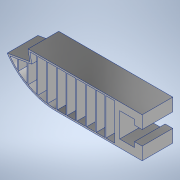
# Autodesk Inventor part: Finray_9_Kerbe_10deg
Saved by Autodesk Inventor 2022 (Build 260153000, 153)
## iProperties
Created: 2022-02-28
Part Number: Finray_9_Kerbe_10deg
Material: Generic
Document SubType Name: Modeling
Designer: richa
Density: 1 g/cm^3
Appearance: Aluminum - Flat
Author: richa
Autodesk Inventor part; units mm, degrees
ref_plane "YZ Plane" through (0, 0, 0) normal (1, 0, 0) x (0, 1, 0)
ref_plane "XZ Plane" through (0, 0, 0) normal (0, 1, 0) x (-1, 0, 0)
ref_plane "XY Plane" through (0, 0, 0) normal (0, 0, 1) x (1, 0, 0)
sketch "Sketch5" plane through (0, 0, 0) normal (0, 0, 1) x (1, 0, 0)
  line L0 (52.8, -15.6) -> (52.8, -10.6)
  line L1 (52.8, -10.6) -> (49.8, -10.6)
  line L2 (49.8, -10.6) -> (49.8, -12.6)
  line L3 (44, -12.6) -> (44, -3)
  line L4 (49.8, -3) -> (49.8, -5)
  line L5 (49.8, -5) -> (52.8, -5)
  line L6 (52.8, -5) -> (52.8, 0)
  line L7 (52.8, 0) -> (7.8, 0)
  line L8 (44, -3) -> (49.8, -3)
  line L9 (44, -12.6) -> (49.8, -12.6)
  line L10 (52.8, -15.6) -> (7.8, -15.6)
  line L11 (7.8, -15.6) -> (0, -15.6)
  line L12 (0, -15.6) -> (0, 0)
  line L13 (0, 0) -> (7.8, 0)
  point P0 (7.8, 0)
  dimension "d41" = 5.8
  dimension "d48" = 44
  dimension "d50" = 3
  dimension "d63" = 45
  dimension "d71" = 0
  dimension "d87" = 5.6
  dimension "d88" = 9.6
  dimension "d97" = 15.6
  constraints: 28 end point, 8 perpendicular, 4 collinear, 3 parallel, 2 horizontal, 1 vertical
  measures "d41" distance between parallel lines of L2 L3
  measures "d48" distance from line of L3 L12.end
  measures "d50" distance of L4.end L5.end
  measures "d63" distance of L0.start L10.end
  measures "d71" distance from line of L12.end L7
  measures "d87" distance from line of L0.end L5
  measures "d88" distance of L3.start L3.end
  measures "d97" distance of L11.end L12.end
extrude "Extrusion2" add sketch "Sketch5" along normal blind 12
sketch "Sketch8" plane through (0, 0, 0) normal (0, 0, -1) x (-1, 0, 0)
  line L0 (-8.1687, 0) -> (-8.8633, -3.9392)
  line L1 (-7.8, 0) -> (-1.143, 0) construction
  line L2 (0, -5.5021) -> (-8.8633, -3.9392)
  line L3 (-7.8, 0) -> (-8.1687, 0)
  line L4 (0, 0) -> (0, -15.6) projected
  line L5 (-52.8, 0) -> (0, 0) projected
  line L6 (-7.8, 0) -> (0, 0)
  line L7 (0, 0) -> (0, -5.5021)
  dimension "d80" = 100
  dimension "d95" = 4
  dimension "d96" = 9
  constraints: 12 end point, 2 collinear, 2 perpendicular, 1 horizontal, 1 point on line
  measures "d80" angle of L0 L1
  measures "d95" distance of L0.start L0.end
  measures "d96" distance of L2.start L0.end
extrude "Extrusion5" cut sketch "Sketch8" against normal through all
fillet "Fillet2" radius 23 1 edges at (0, -15.6, 6)
shell "Shell1" thickness 0.62 removed faces 1 at (23.9679, -7.5131, 12)
sketch "Sketch13" plane through (0, 0, 12) normal (0, 0, 1) x (1, 0, 0)
  line L0 (19.0404, -15.6) -> (52.8, -15.6) projected
  line L1 (42.0526, -15.6) -> (42.0526, 0)
  line L2 (52.8, 0) -> (8.1687, 0) projected
  line L3 (52.8, 0) -> (8.1687, 0) projected
  line L4 (52.8, -5) -> (52.8, 0) projected
  line L5 (49.8, -5) -> (52.8, -5) projected
  line L6 (49.8, -3) -> (49.8, -5) projected
  line L7 (44, -3) -> (49.8, -3) projected
  line L8 (44, -12.6) -> (44, -3) projected
  line L9 (49.8, -12.6) -> (44, -12.6) projected
  line L10 (49.8, -10.6) -> (49.8, -12.6) projected
  line L11 (52.8, -10.6) -> (49.8, -10.6) projected
  line L12 (52.8, -15.6) -> (52.8, -10.6) projected
  line L13 (42.0526, 0) -> (52.8, 0)
  line L14 (52.8, -5) -> (52.8, 0) projected
  line L15 (52.8, -5) -> (52.8, 0)
  line L16 (52.8, 0) -> (52.8, -5)
  line L17 (44, -12.6) -> (44, -3) projected
  line L18 (44, -3) -> (44, -12.6)
  line L19 (49.8, -12.6) -> (44, -12.6) projected
  line L20 (44, -12.6) -> (49.8, -12.6)
  line L21 (43.38, -13.22) -> (50.42, -13.22) projected
  line L22 (52.8, -10.6) -> (52.8, -15.6)
  line L23 (52.8, -15.6) -> (42.0526, -15.6)
  line L24 (44, -3) -> (49.8, -3) projected
  line L25 (44, -3) -> (49.8, -3)
  line L26 (49.8, -3) -> (49.8, -5)
  line L27 (49.8, -5) -> (52.8, -5)
  line L28 (52.8, -10.6) -> (49.8, -10.6)
  line L29 (49.8, -10.6) -> (49.8, -12.6)
  point P0 (0, 0)
  dimension "d102" = 10.7474
  constraints: 26 end point, 10 collinear, 2 point on line, 2 vertical, 1 parallel
  measures "d102" distance between parallel lines of L4 L1
extrude "Extrusion7" add sketch "Sketch13" against normal blind 12
sketch "Sketch14" plane through (8.9076, -0.62, 0.62) normal (0, 0, 1) x (1, 0, 0)
  line L0 (33.145, -14.36) -> (33.145, 0) projected
  line L1 (33.145, 0) -> (0, 0) projected
  line L2 (0.6739, -3.8221) -> (0, 0) projected
  line L3 (-7.835, -5.3225) -> (0.6739, -3.8221) projected
  arc A0 (-7.835, -5.3225) -> (10.1328, -14.36) centre (10.1328, 8.02) ccw projected
  line L4 (10.1328, -14.36) -> (33.145, -14.36) projected
  point P0 (-8.9076, 0.62)
extrude "Extrusion8" cut sketch "Sketch14" against normal blind 12
sketch "Sketch15" plane through (0, 0, 12) normal (0, 0, 1) x (1, 0, 0)
  line L0 (42.0526, -0.62) -> (8.9076, -0.62) construction
  line L1 (19.0404, -14.98) -> (42.0526, -14.98) projected
  line L2 (38.2426, -0.62) -> (38.6226, -0.62)
  line L3 (38.6226, -0.62) -> (38.6226, -14.98)
  line L4 (38.6226, -14.98) -> (38.2426, -14.98)
  line L5 (38.2426, -14.98) -> (38.2426, -0.62)
  line L6 (34.4326, -0.62) -> (34.8126, -0.62)
  line L7 (34.8126, -0.62) -> (34.8126, -14.98)
  line L8 (34.8126, -14.98) -> (34.4326, -14.98)
  line L9 (34.4326, -14.98) -> (34.4326, -0.62)
  line L10 (30.6226, -0.62) -> (31.0026, -0.62)
  line L11 (31.0026, -0.62) -> (31.0026, -14.98)
  line L12 (31.0026, -14.98) -> (30.6226, -14.98)
  line L13 (30.6226, -14.98) -> (30.6226, -0.62)
  line L14 (26.8126, -0.62) -> (27.1926, -0.62)
  line L15 (27.1926, -0.62) -> (27.1926, -14.98)
  line L16 (27.1926, -14.98) -> (26.8126, -14.98)
  line L17 (26.8126, -14.98) -> (26.8126, -0.62)
  line L18 (23.0026, -0.62) -> (23.3826, -0.62)
  line L19 (23.3826, -0.62) -> (23.3826, -14.98)
  line L20 (23.3826, -14.98) -> (23.0026, -14.98)
  line L21 (23.0026, -14.98) -> (23.0026, -0.62)
  line L22 (19.1926, -0.62) -> (19.5726, -0.62)
  line L23 (19.5726, -0.62) -> (19.5726, -14.98)
  line L24 (19.5726, -14.98) -> (19.1926, -14.98)
  line L25 (19.1926, -14.98) -> (19.1926, -0.62)
  line L26 (15.3826, -0.62) -> (15.7626, -0.62)
  line L27 (15.7626, -0.62) -> (15.7626, -14.98)
  line L28 (15.7626, -14.98) -> (15.3826, -14.98)
  line L29 (15.3826, -14.98) -> (15.3826, -0.62)
  line L30 (11.5726, -0.62) -> (11.9526, -0.62)
  line L31 (11.9526, -0.62) -> (11.9526, -14.4807)
  line L32 (11.5726, -14.3539) -> (11.5726, -0.62)
  arc A0 (1.0726, -5.9425) -> (19.0404, -14.98) centre (19.0404, 7.4) ccw projected
  line L33 (42.0526, -0.62) -> (42.0526, -14.98) projected
  line L34 (1.0726, -5.9425) -> (9.5815, -4.4421) projected
  arc A1 (0, -5.5021) -> (19.0404, -15.6) centre (19.0404, 7.4) ccw projected
  line L35 (4.3326, -5.3677) -> (3.9526, -5.3677)
  line L36 (3.9526, -5.3677) -> (3.9526, -9.9597)
  line L37 (3.9526, -9.9597) -> (4.3326, -9.9597)
  line L38 (4.3326, -9.9597) -> (4.3326, -5.3677)
  line L39 (8.1426, -4.6475) -> (7.7626, -4.6475)
  line L40 (7.7626, -4.6475) -> (7.7626, -12.5934)
  line L41 (7.7626, -12.5934) -> (8.1426, -12.5934)
  line L42 (8.1426, -12.5934) -> (8.1426, -4.6475)
  point P0 (0, 0)
  point P1 (11.5726, -13.6973)
  point P2 (11.9526, -13.828)
  dimension "d105" = 0.38
  dimension "d106" = 3.81
  dimension "d107" = 0.38
  dimension "d108" = 0.38
  dimension "d109" = 0.38
  dimension "d110" = 0.38
  dimension "d111" = 0.38
  dimension "d112" = 0.38
  dimension "d113" = 0.38
  dimension "d116" = 3.81
  dimension "d117" = 3.81
  dimension "d118" = 0.38
  dimension "d119" = 0.38
  dimension "d120" = 3.81
  dimension "d121" = 3.81
  dimension "d122" = 3.81
  dimension "d123" = 3.81
  dimension "d124" = 3.81
  dimension "d125" = 3.81
  dimension "d126" = 3.81
  constraints: 78 end point, 19 parallel, 16 point on line, 10 horizontal, 10 perpendicular, 3 point on circle
  measures "d105" distance between parallel lines of L3 L5
  measures "d106" distance between parallel lines of L33 L5
  measures "d107" distance between parallel lines of L7 L9
  measures "d108" distance of L10.start L10.end
  measures "d109" distance of L14.start L14.end
  measures "d110" distance between parallel lines of L19 L21
  measures "d111" distance between parallel lines of L23 L25
  measures "d112" distance between parallel lines of L27 L29
  measures "d113" distance between parallel lines of L31 L32
  measures "d116" distance between parallel lines of L5 L9
  measures "d117" distance between parallel lines of L9 L13
  measures "d118" distance of L39.start L39.end
  measures "d119" distance of L35.start L35.end
  measures "d120" distance between parallel lines of L13 L17
  measures "d121" distance between parallel lines of L17 L21
  measures "d122" distance between parallel lines of L21 L25
  measures "d123" distance between parallel lines of L25 L29
  measures "d124" distance between parallel lines of L29 L32
  measures "d125" distance between parallel lines of L32 L40
  measures "d126" distance between parallel lines of L40 L36
extrude "Extrusion9" add sketch "Sketch15" against normal blind 12 contours L25 L22 L23 L1 | L21 L18 L19 L1 | L17 L14 L15 L1 | L13 L10 L11 L1 | L9 L6 L7 L1 | L5 L2 L3 L1 | L26 L27 A0 L29 | A0 L27 L28 L29 | L30 L31 A0 L32 | L42 L41 L40 A0 | A0 L40 L34 L42 | L36 A0 L38 L37 | L34 L40 L39 L42 | L36 L34 L38 A0 | L36 L35 L34
equation "\"l1\" = 8"
equation "\"d1\" = 0.38"
body "Solid2"
